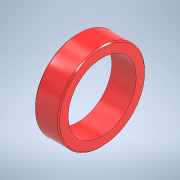
# Autodesk Inventor part: Проставка
Saved by Autodesk Inventor 2021 (Build 250183000, 183)
## iProperties
Created: 2023-04-15
Part Number: Проставка
Material: Сталь, углеродистая
Document SubType Name: Modeling
Designer: gdevc
Density: 7.85 g/cm^3
Appearance: Светло-красный
Author: gdevc
Autodesk Inventor part; units mm, degrees
ref_plane "YZ Plane" through (0, 0, 0) normal (1, 0, 0) x (0, 1, 0)
ref_plane "XZ Plane" through (0, 0, 0) normal (0, 1, 0) x (-1, 0, 0)
ref_plane "XY Plane" through (0, 0, 0) normal (0, 0, 1) x (1, 0, 0)
sketch "Эскиз1" plane through (0, 0, 0) normal (0, 0, 1) x (1, 0, 0)
  line L0 (0, 9) -> (5, 9)
  line L1 (5, 9) -> (5, 7)
  line L2 (5, 7) -> (0, 7)
  line L3 (0, 7) -> (0, 9)
  line L4 (0, 0) -> (5.6072, 0)
  dimension "d0" = 14
  dimension "d1" = 2
  dimension "d2" = 5
  constraints: 10 end point, 2 horizontal, 2 parallel, 1 perpendicular, 1 point on line
  measures "d0" diameter of L2 L4
  measures "d1" distance between parallel lines of L2 L0
  measures "d2" distance between parallel lines of L1 L3
revolve "Вращение1" add sketch "Эскиз1" angle 360 about axis through (0, 0, 0) along (1, 0, 0)
chamfer "Фаска1" distance 0.25 angle 45 2 edges at (5, -9, 0) (0, -9, 0)
